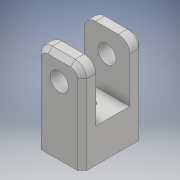
# Autodesk Inventor part: cylinder clevis
Saved by Autodesk Inventor 2017 (Build 210142000, 142)
## iProperties
Created: 2017-12-08
Part Number: cylinder clevis
Material: Generic
Document SubType Name: Modeling
Designer: RLanting
Density: 1 g/cm^3
Appearance: Default
Author: RLanting
Autodesk Inventor part; units mm, degrees
ref_plane "YZ Plane" through (0, 0, 0) normal (1, 0, 0) x (0, 1, 0)
ref_plane "XZ Plane" through (0, 0, 0) normal (0, 1, 0) x (-1, 0, 0)
ref_plane "XY Plane" through (0, 0, 0) normal (0, 0, 1) x (1, 0, 0)
sketch "Sketch1" plane through (0, 0, 0) normal (0, 0, 1) x (1, 0, 0)
  line L0 (10, -7.5) -> (-10, -7.5)
  line L1 (-10, -7.5) -> (-10, 7.5)
  line L2 (-10, 7.5) -> (10, 7.5)
  line L3 (10, 7.5) -> (10, -7.5)
  line L4 (10, -7.5) -> (-10, 7.5) construction
  line L5 (-10, -7.5) -> (10, 7.5) construction
  line L6 (-10, 7.5) -> (10, 7.5)
  line L7 (10, 7.5) -> (10, 13.5)
  line L8 (10, 13.5) -> (-10, 13.5)
  line L9 (-10, 13.5) -> (-10, 7.5)
  line L10 (-10, -7.5) -> (10, -7.5)
  line L11 (10, -7.5) -> (10, -13.5)
  line L12 (10, -13.5) -> (-10, -13.5)
  line L13 (-10, -13.5) -> (-10, -7.5)
  point P0 (0, 0)
  dimension "d0" = 15
  dimension "d1" = 20
  dimension "d2" = 6
  constraints: 28 end point, 7 equal length, 4 perpendicular, 2 midpoint, 1 collinear, 1 horizontal
  measures "d0" distance between parallel lines of L0 L2
  measures "d1" distance between parallel lines of L3 L1
  measures "d2" distance between parallel lines of L2 L8
extrude "Extrusion1" add sketch "Sketch1" against normal blind 15
extrude "Extrusion2" add sketch "Sketch1" along normal blind 25 contours L11 L12 L13 L0 | L2 L9 L8 L7
sketch "Sketch2" plane through (-10, 13.5, -15) normal (0, 1, 0) x (1, 0, 0)
  line L0 (20, -15) -> (0, -15) projected
  line L1 (20, -40) -> (0, -40) construction
  line L2 (10, -40) -> (10, -30) construction
  circle A0 centre (10, -30) radius 4
  point P0 (10, -15)
  dimension "d7" = 8
  dimension "d8" = 10
  constraints: 2 end point, 1 centre point, 1 coincident, 1 midpoint, 1 vertical
  measures "d7" diameter of A0
  measures "d8" distance of L2.start L2.end
extrude "Extrusion3" cut sketch "Sketch2" against normal through all
fillet "Fillet1" radius 5 4 edges at (-10, 10.5, 25) (10, 10.5, 25) (-10, -10.5, 25) (10, -10.5, 25)
sketch "Sketch3" plane through (0, 0, -15) normal (0, 0, -1) x (-1, 0, 0)
  circle A0 centre (0, 0) radius 2.15
  dimension "d12" = 4.3
  constraints: 1 centre point, 1 coincident
  measures "d12" diameter of A0
extrude "Extrusion4" cut sketch "Sketch3" against normal through all
chamfer "Chamfer1" distance 2 angle 45 10 edges at (10, 13.5, 2.5) (8.5355, 13.5, 23.5355) (0, 13.5, 25) (-8.5355, 13.5, 23.5355) (-10, 13.5, 2.5) (10, -13.5, 2.5) (8.5355, -13.5, 23.5355) (0, -13.5, 25) (-8.5355, -13.5, 23.5355) (-10, -13.5, 2.5)
body "Solid1"
